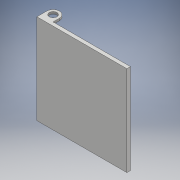
# Autodesk Inventor part: MecanumPlate_FEA
Saved by Autodesk Inventor 2018 (Build 220112000, 112)
## iProperties
Created: 2017-09-19
Part Number: MecanumPlate_FEA
Material: Generic
Document SubType Name: Modeling
Designer: P136265
Density: 1 g/cm^3
Appearance: Default
Author: P136265
Autodesk Inventor part; units mm, degrees
ref_plane "YZ Plane" through (0, 0, 0) normal (1, 0, 0) x (0, 1, 0)
ref_plane "XZ Plane" through (0, 0, 0) normal (0, 1, 0) x (-1, 0, 0)
sketch "Sketch1" plane through (0, 0, 0) normal (0, 0, 1) x (1, 0, 0)
  line L0 (-250, -10) -> (250, -10)
  line L1 (250, -10) -> (250, 10)
  line L2 (250, 10) -> (-250, 10)
  line L3 (-250, 10) -> (-250, -10)
  line L4 (-250, -10) -> (250, 10) construction
  line L5 (250, -10) -> (-250, 10) construction
  point P0 (0, 0)
  dimension "d0" = 500
  dimension "d1" = 20
  constraints: 12 end point, 2 midpoint, 2 parallel, 1 horizontal, 1 perpendicular
  measures "d0" distance of L2.end L1.end
  measures "d1" distance of L1.end L0.end
extrude "Extrusion1" add sketch "Sketch1" along normal mid plane 500
sketch "Sketch2" plane through (0, 0, 250) normal (0, 0, 1) x (1, 0, 0)
  arc A0 (-180, 45) -> (-250, 45) centre (-215, 45) ccw
  line L0 (250, 10) -> (-250, 10) construction
  circle A1 centre (-215, 45) radius 21
  line L1 (-250, 45) -> (-250, 0)
  line L2 (-180, 45) -> (-180, 0)
  line L3 (-180, 0) -> (-250, 0)
  point P0 (0, 0)
  dimension "d4" = 70
  dimension "d5" = 215
  dimension "d6" = 45
  dimension "d7" = 42
  dimension "d9" = 10
  constraints: 6 end point, 2 centre point, 2 point on circle, 2 tangent, 2 vertical, 1 coincident, 1 perpendicular
  measures "d4" diameter of A0
  measures "d5" horizontal distance of point (0, 0) A0.centre
  measures "d6" vertical distance of point (0, 0) A0.centre
  measures "d7" diameter of A1
  measures "d9" distance between parallel lines of L3 L0
extrude "Extrusion2" add sketch "Sketch2" against normal blind 12
ref_plane "Work Plane1" through (0, 0, 85) normal (0, 0, 1) x (1, 0, 0)
sketch "Sketch3" plane through (0, 0, 85) normal (0, 0, 1) x (1, 0, 0)
  arc A0 (-180, 45) -> (-250, 45) centre (-215, 45) ccw construction
  circle A1 centre (-215, 45) radius 21 construction
  line L0 (-180, 45) -> (-180, 10) construction
  line L1 (-250, 45) -> (-250, -10) construction
  circle A2 centre (-215, 45) radius 21
  arc A3 (-180, 45) -> (-250, 45) centre (-215, 45) ccw
  line L2 (-250, 45) -> (-250, 0)
  line L3 (-180, 45) -> (-180, 0)
  line L4 (-180, 0) -> (-250, 0)
  point P0 (0, 0)
  constraints: 6 end point, 4 tangent, 3 point on line, 2 centre point, 2 coincident, 2 concentric, 2 point on circle, 1 perpendicular
extrude "Extrusion3" add sketch "Sketch3" along normal blind 12
body "Solid1"
